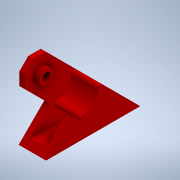
# Autodesk Inventor part: WeaponMountV1
Saved by Autodesk Inventor 2020 (Build 240168000, 168)
## iProperties
Created: 2024-02-06
Part Number: WeaponMountV1
Material: PETG
Document SubType Name: Modeling
Designer: smz3rm
Density: 1 g/cm^3
Appearance: Generic
Author: smz3rm
Autodesk Inventor part; units mm, degrees
ref_plane "YZ Plane" through (0, 0, 0) normal (1, 0, 0) x (0, 1, 0)
ref_plane "XZ Plane" through (0, 0, 0) normal (0, 1, 0) x (-1, 0, 0)
ref_plane "XY Plane" through (0, 0, 0) normal (0, 0, 1) x (1, 0, 0)
sketch "Sketch1" plane through (0, 0, 0) normal (1, 0, 0) x (0, 1, 0)
  line L0 (0, 0) -> (30, -30)
  line L1 (30, -30) -> (0, -30)
  line L2 (0, -30) -> (0, 0)
  circle A0 centre (52.45, -14.45) radius 2.5
  line L3 (66.35, -8.6924) -> (66.35, -20.2076)
  line L4 (66.35, -20.2076) -> (58.2076, -28.35)
  line L5 (58.2076, -28.35) -> (46.6924, -28.35)
  line L6 (46.6924, -28.35) -> (38.55, -20.2076)
  line L7 (38.55, -20.2076) -> (38.55, -8.6924)
  line L8 (38.55, -8.6924) -> (46.6924, -0.55)
  line L9 (46.6924, -0.55) -> (58.2076, -0.55)
  line L10 (58.2076, -0.55) -> (66.35, -8.6924)
  line L11 (38.55, -8.6924) -> (23.6212, -23.6212)
  line L12 (58.2076, -28.35) -> (0, -86.5576)
  line L13 (0, -86.5576) -> (0, -30)
  point P0 (0, -30)
  dimension "d0" = 45
  dimension "d1" = 30
  dimension "d2" = 5
  dimension "d4" = 13.9
  dimension "d10" = 52.45
  dimension "d12" = 14.45
  constraints: 28 end point, 2 collinear, 2 horizontal, 2 perpendicular, 1 centre point, 1 coincident, 1 point on line, 1 vertical, 17 other
  measures "d0" angle of L2 L0
  measures "d1" distance of L0.end L1.end
  measures "d2" diameter of A0
  measures "d4" distance from line of L9 A0.centre
  measures "d10" distance from line of L2 A0.centre
  measures "d12" vertical distance of A0.centre L0.start
extrude "Extrusion1" add sketch "Sketch1" along normal blind 5
sketch "Sketch2" plane through (5, 0, 0) normal (1, 0, 0) x (0, 0, -1)
  line L0 (20.2076, 66.35) -> (8.6924, 66.35) projected
  line L1 (23.6212, 23.6212) -> (0, 0) projected
  circle A0 centre (14.45, 52.45) radius 2.5 projected
  line L2 (5, 5) -> (81.5576, 5)
  line L3 (8.6924, 66.35) -> (0.55, 58.2076) projected
  line L4 (0.55, 58.2076) -> (0.55, 46.6924) projected
  line L5 (86.5576, 0) -> (20.2076, 66.35) projected
  line L6 (0.55, 46.6924) -> (23.6212, 23.6212) projected
  line L7 (0, 0) -> (86.5576, 0) projected
  point P0 (81.699, 4)
  dimension "d28" = 5
  constraints: 2 end point, 2 point on line, 1 horizontal
  measures "d28" distance between parallel lines of L7 L2
extrude "Extrusion2" add sketch "Sketch2" along normal blind 15 contours L5 L7 L1 L2
sketch "Sketch3" plane through (5, 0, 0) normal (1, 0, 0) x (0, 0, -1)
  line L0 (81.5576, 5) -> (20.2076, 66.35) projected
  line L1 (20.2076, 66.35) -> (8.6924, 66.35) projected
  line L2 (8.6924, 66.35) -> (0.55, 58.2076) projected
  line L3 (0.55, 58.2076) -> (0.55, 46.6924) projected
  line L4 (0.55, 46.6924) -> (23.6212, 23.6212) projected
  line L5 (23.6212, 23.6212) -> (5, 5) projected
  circle A0 centre (14.45, 52.45) radius 2.5 projected
  line L6 (5, 5) -> (81.5576, 5) projected
  circle A1 centre (14.45, 52.45) radius 2.5 projected
  circle A2 centre (14.45, 52.45) radius 3.65
  circle A3 centre (14.45, 52.45) radius 6.5
  point P0 (0, 0)
  dimension "d14" = 7.3
  dimension "d15" = 13
  constraints: 2 centre point, 2 coincident
  measures "d14" diameter of A2
  measures "d15" diameter of A3
extrude "Extrusion3" add sketch "Sketch3" along normal blind 6 contours A3
ref_plane "Work Plane1" through (12.5, 0, 0) normal (1, 0, 0) x (0, 0, -1)
mirror "Mirror1" about plane through (12.5, 0, 0) normal (1, 0, 0) of "Extrusion1"
sketch "Sketch4" plane through (25, 46.6924, -0.55) normal (1, 0, 0) x (0, 0, -1)
  circle A0 centre (13.9, 5.7576) radius 2.5 projected
  circle A1 centre (13.9, 5.7576) radius 13.9
  line L0 (8.1424, 19.6576) -> (0, 11.5151) projected
  line L1 (0, 11.5151) -> (0, 0) projected
  line L2 (0, 0) -> (23.0712, -23.0712) projected
  line L3 (23.0712, -23.0712) -> (-0.55, -46.6924) projected
  line L4 (86.0076, -46.6924) -> (19.6576, 19.6576) projected
  line L5 (19.6576, 19.6576) -> (8.1424, 19.6576) projected
  circle A2 centre (13.9, 5.7576) radius 2.5 projected
  line L6 (-0.55, -46.6924) -> (86.0076, -46.6924) projected
  point P0 (4.0712, -4.0712)
  point P1 (23.7288, 15.5864)
  dimension "d19" = 27.8
  constraints: 1 centre point, 1 coincident
  measures "d19" diameter of A1
extrude "Extrusion4" cut sketch "Sketch4" against normal up to surface (5 mm away) contours A0 | A1 | A1 L5 L4 | L2 L1 A1 | A1 L0 L5 | L1 L0 A1
sketch "Sketch5" plane through (25, 0, 0) normal (1, 0, 0) x (0, 0, -1)
  circle A0 centre (14.45, 52.45) radius 6.5 projected
  arc A1 (14.7256, 36.0523) -> (30.8477, 52.1744) centre (14.45, 52.45) ccw construction
  arc A2 (14.7677, 33.5527) -> (33.3473, 52.1323) centre (14.45, 52.45) ccw
  arc A3 (14.6836, 38.552) -> (28.348, 52.2164) centre (14.45, 52.45) ccw
  arc A4 (14.6836, 38.552) -> (14.7677, 33.5527) centre (14.7256, 36.0523) ccw
  arc A5 (33.3473, 52.1323) -> (28.348, 52.2164) centre (30.8477, 52.1744) ccw
  line L0 (4.6212, 42.6212) -> (23.6212, 23.6212) projected
  line L1 (86.5576, 0) -> (24.2788, 62.2788) projected
  arc A6 (4.6212, 42.6212) -> (24.2788, 62.2788) centre (14.45, 52.45) ccw projected
  point P0 (0, 0)
  point P1 (32.6155, 53.9421)
  point P2 (12.9579, 34.2845)
  point P3 (0.55, 46.6924)
  point P4 (20.2076, 66.35)
  dimension "d22" = 13.9
  dimension "d23" = 5
  constraints: 10 point on circle, 6 tangent, 5 centre point, 1 coincident
  measures "d22" radius of A3
  measures "d23" radial gap between concentric circles of A3 A2
extrude "Extrusion5" cut sketch "Sketch5" against normal up to surface (5 mm away) contours L0 A6 A4 | A5 A6 L1
extrude "Extrusion6" add sketch "Sketch5" along normal blind 19.5 contours A4 A3 A5 A2
equation "\"d0\" = FrontAngle"
equation "\"d1\" = Height"
equation "\"d4\" = 0.5 * WeaponMotorDia"
equation "\"d10\" = WeaponHeight + WeaponMountThickness"
equation "\"d12\" = 0.5 * WeaponDia - WeaponBite"
equation "\"d5\" = WeaponMountThickness"
equation "\"d28\" = WeaponMountThickness"
equation "\"d8\" = WeaponOpeningWidth"
equation "\"d19\" = WeaponMotorDia"
equation "\"d22\" = 0.5 * WeaponMotorDia"
equation "\"d23\" = WeaponMountThickness"
equation "\"d24\" = WeaponMountThickness"
equation "\"d26\" = -0.5 * WeaponOpeningWidth + WeaponCenterToMotorBack - WeaponMountThickness"
equation "\"WeaponDia\" = 88.9"
equation "\"d18\" = 0.5 * WeaponOpeningWidth"
equation "\"WeaponMotorDia\" = 27.8"
equation "\"FrontAngle\" = 45deg"
equation "\"Height\" = 30"
equation "\"WeaponHeight\" = 47.45"
equation "\"WeaponMountThickness\" = 5"
equation "\"WeaponBite\" = 30"
equation "\"WeaponOpeningWidth\" = 15"
equation "\"WeaponCenterToMotorBack\" = 32"
body "Solid1"
